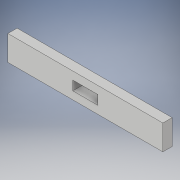
# Autodesk Inventor part: mobile_table_bottom
Saved by Autodesk Inventor 2019.4 (Build 234330000, 330)
## iProperties
Created: 2019-12-14
Part Number: mobile_table_bottom
Material: Generic
Document SubType Name: Modeling
Designer: fabfarm
Density: 1 g/cm^3
Appearance: Default
Author: fabfarm
Autodesk Inventor part; units mm, degrees
ref_plane "YZ Plane" through (0, 0, 0) normal (1, 0, 0) x (0, 1, 0)
ref_plane "XZ Plane" through (0, 0, 0) normal (0, 1, 0) x (-1, 0, 0)
ref_plane "XY Plane" through (0, 0, 0) normal (0, 0, 1) x (1, 0, 0)
sketch "Sketch1" plane through (0, 0, 0) normal (0, 0, 1) x (1, 0, 0)
  line L0 (0, 0) -> (310, 0)
  line L1 (310, 0) -> (310, 50)
  line L2 (310, 50) -> (0, 50)
  line L3 (0, 50) -> (0, 0)
  dimension "d0" = 310
  dimension "d1" = 50
  constraints: 8 end point, 2 parallel, 1 horizontal, 1 perpendicular
  measures "d0" distance of L1.end L2.end
  measures "d1" distance of L0.end L1.end
extrude "Extrusion1" add sketch "Sketch1" along normal blind 18.55
sketch "Sketch2" plane through (0, 0, 18.55) normal (0, 0, 1) x (1, 0, 0)
  line L0 (130, 34.3) -> (180, 34.3)
  line L1 (180, 34.3) -> (180, 15.7)
  line L2 (180, 15.7) -> (130, 15.7)
  line L3 (130, 15.7) -> (130, 34.3)
  line L4 (130, 25) -> (0, 25) construction
  line L5 (0, 50) -> (0, 0) projected
  line L6 (180, 25) -> (310, 25) construction
  line L7 (310, 0) -> (310, 50) projected
  dimension "d4" = 18.6
  dimension "d5" = 50
  constraints: 12 end point, 4 midpoint, 3 horizontal, 2 parallel, 1 collinear, 1 perpendicular
  measures "d4" distance between parallel lines of L0 L2
  measures "d5" distance of L1.end L2.end
extrude "Extrusion2" cut sketch "Sketch2" against normal blind 20
body "Solid1"
